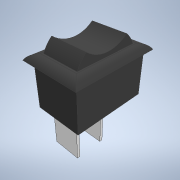
# Autodesk Inventor part: Выключатель маленький
Saved by Autodesk Inventor 2021.1 (Build 251245010, 245A)
## iProperties
Created: 2022-11-29
Part Number: Выключатель маленький
Material: Типовые
Document SubType Name: Modeling
Designer: Andrew
Density: 1 g/cm^3
Appearance: По умолчанию
Author: Andrew
Autodesk Inventor part; units mm, degrees
ref_plane "YZ Plane" through (0, 0, 0) normal (1, 0, 0) x (0, 1, 0)
ref_plane "XZ Plane" through (0, 0, 0) normal (0, 1, 0) x (-1, 0, 0)
ref_plane "XY Plane" through (0, 0, 0) normal (0, 0, 1) x (1, 0, 0)
sketch "Эскиз1" plane through (0, 0, 0) normal (0, 1, 0) x (-1, 0, 0)
  line L0 (6, 14) -> (-2.4, 14)
  line L1 (-2.4, 14) -> (-2.4, 0.8)
  line L2 (-2.4, 0.8) -> (6, 0.8)
  line L3 (6, 0.8) -> (6, 14)
  point P0 (0, 0)
  dimension "d0" = 8.4
  dimension "d1" = 13.2
  constraints: 8 end point, 2 parallel, 1 horizontal, 1 perpendicular
  measures "d0" distance of L2.end L1.end
  measures "d1" distance of L1.end L0.end
extrude "Выдавливание1" add sketch "Эскиз1" along normal blind 8
sketch "Эскиз2" plane through (0, 8, 0) normal (0, 1, 0) x (1, 0, 0)
  line L0 (-7.1, -15) -> (3.4, -15)
  line L1 (3.4, -15) -> (3.4, 0)
  line L2 (3.4, 0) -> (-7.1, 0)
  line L3 (-7.1, 0) -> (-7.1, -15)
  line L4 (-6, -14) -> (2.4, -14) projected
  line L5 (-6, -0.8) -> (-6, -14) projected
  point P0 (0, 0)
  dimension "d4" = 10.5
  dimension "d5" = 15
  dimension "d6" = 1
  dimension "d7" = 1.1
  constraints: 8 end point, 2 parallel, 1 horizontal, 1 perpendicular
  measures "d4" distance of L2.end L1.end
  measures "d5" distance of L1.end L0.end
  measures "d6" distance between parallel lines of L4 L0
  measures "d7" distance between parallel lines of L5 L3
extrude "Выдавливание2" add sketch "Эскиз2" along normal blind 1
fillet "Сопряжение1" radius 2 4 edges at (-1.85, 9, 15) (3.4, 9, 7.5) (-1.85, 9, 0) (-7.1, 9, 7.5)
sketch "Эскиз3" plane through (0, 9, 0) normal (0, 1, 0) x (1, 0, 0)
  line L0 (-5.0869, -12.9218) -> (1.4131, -12.9218)
  line L1 (1.4131, -12.9218) -> (1.4131, -2.2574)
  line L2 (1.4131, -2.2574) -> (-5.0869, -2.2574)
  line L3 (-5.0869, -2.2574) -> (-5.0869, -12.9218)
  line L4 (-5.3679, -13.2679) -> (-5.3679, -1.7321) projected
  point P0 (0, 0)
  dimension "d12" = 6.5
  constraints: 8 end point, 2 parallel, 1 perpendicular
  measures "d12" distance of L1.end L2.end
extrude "Выдавливание3" add sketch "Эскиз3" along normal blind 2
sketch "Эскиз4" plane through (1.4131, 9, 12.9218) normal (1, 0, 0) x (0, 0, -1)
  arc A0 (1.5475, 2) -> (9.1169, 2) centre (5.3322, -2.5272) ccw
  line L0 (0, 0) -> (0, 2)
  line L1 (0, 2) -> (1.5475, 2)
  line L2 (10.6644, 0) -> (10.6644, 2) projected
  line L3 (9.1169, 2) -> (10.6644, 2)
  arc A1 (1.5475, 2) -> (9.1169, 2) centre (5.3322, 6.6369) ccw
  line L4 (1.5475, 2) -> (9.1169, 2)
  line L5 (10.6644, 2) -> (0, 2) projected
  point P0 (12.9218, -9)
  constraints: 8 end point, 6 point on circle, 2 centre point, 1 collinear, 1 perpendicular, 1 point on line
extrude "Выдавливание4" cut sketch "Эскиз4" against normal through all contours A0 L0 L1 | L4 A1 | L3 L2 A0
sketch "Эскиз5" plane through (0, 0, 0) normal (0, -1, 0) x (1, 0, 0)
  line L0 (0.6293, 12.6934) -> (-4.3707, 12.6934)
  line L1 (-4.3707, 12.6934) -> (-4.3707, 12.1934)
  line L2 (-4.3707, 12.1934) -> (0.6293, 12.1934)
  line L3 (0.6293, 12.1934) -> (0.6293, 12.6934)
  line L4 (0.6293, 7.6934) -> (-4.3707, 7.6934)
  line L5 (-4.3707, 7.6934) -> (-4.3707, 7.1934)
  line L6 (-4.3707, 7.1934) -> (0.6293, 7.1934)
  line L7 (0.6293, 7.1934) -> (0.6293, 7.6934)
  point P0 (0, 0)
  dimension "d18" = 5
  dimension "d19" = 0.5
  dimension "d22" = 5
  constraints: 16 end point, 2 parallel, 1 collinear, 1 horizontal, 1 perpendicular, 1 vertical, 7 other
  measures "d18" distance of L2.end L1.end
  measures "d19" distance of L1.end L0.end
  measures "d22" distance of L0.start L4.start
extrude "Выдавливание5" add sketch "Эскиз5" along normal blind 7 separate body
